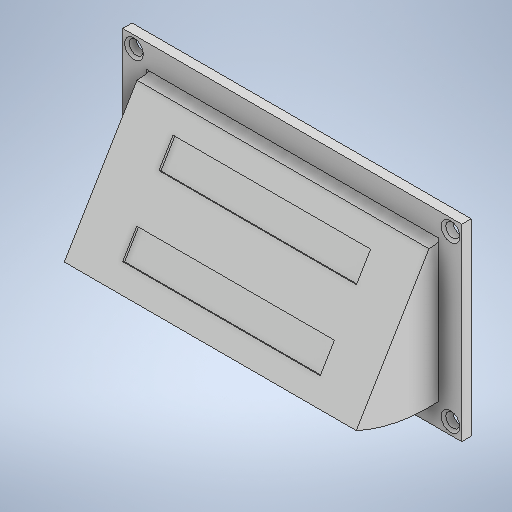
# Autodesk Inventor part: DsholdtilterV1
Saved by Autodesk Inventor 2025.1 (Build 291241000, 241)
## iProperties
Created: 2024-09-22
Part Number: DsholdtilterV1
Material: Generic
Document SubType Name: Modeling
Designer: ishaa
Density: 1 g/cm^3
Appearance: Default
Author: ishaa
Autodesk Inventor part; units mm, degrees
ref_plane "YZ Plane" through (0, 0, 0) normal (1, 0, 0) x (0, 1, 0)
ref_plane "XZ Plane" through (0, 0, 0) normal (0, 1, 0) x (-1, 0, 0)
ref_plane "XY Plane" through (0, 0, 0) normal (0, 0, 1) x (1, 0, 0)
sketch "Sketch1" plane through (0, 0, 0) normal (0, 0, 1) x (1, 0, 0)
  line L0 (0, 0) -> (62, 0)
  line L1 (62, 0) -> (62, 30)
  line L2 (62, 30) -> (0, 30)
  line L3 (0, 30) -> (0, 0)
  dimension "d0" = 62
  dimension "d1" = 30
  constraints: 8 end point, 2 parallel, 1 horizontal, 1 perpendicular
  measures "d0" distance of L2.end L1.end
  measures "d1" distance of L1.end L0.end
sketch "Sketch2" plane through (0, 0, 0) normal (1, 0, 0) x (0, 1, 0)
  line L0 (0, 0) -> (30, 0) projected
  arc A0 (16.1062, 11.6791) -> (15, 0) centre (36.6604, 3.8403) ccw
  constraints: 2 point on circle, 1 centre point, 1 midpoint
sweep "Sweep1" add profiles "Sketch1" path "Sketch2" path curves A0
sketch "Sketch3" plane through (62, 0, 0) normal (0, 0, -1) x (-1, 0, 0)
  line L0 (0, 0) -> (0, 30) projected
  line L1 (62, 0) -> (0, 0) projected
  line L2 (62, 30) -> (62, 0) projected
  line L3 (0, 30) -> (62, 30) projected
  line L4 (0, 30) -> (62, 0) construction
  line L5 (0, 0) -> (62, 30) construction
  line L6 (67, 35) -> (67, -5)
  line L7 (67, -5) -> (-5, -5)
  line L8 (-5, -5) -> (-5, 35)
  line L9 (-5, 35) -> (67, 35)
  dimension "d4" = 5
  constraints: 12 end point, 3 other
  measures "d4" distance between parallel lines of L3 L9
extrude "Extrusion1" add sketch "Sketch3" against normal blind 2
sketch "Sketch4" plane through (67, -5, 0) normal (0, 0, -1) x (-1, 0, 0)
  point P0 (67, 5)
sketch "Sketch6" plane through (0, 28.9732, 3.9694) normal (0, 0.514, 0.8578) x (1, 0, 0)
  line L0 (0, 1.893) -> (62, 1.893) construction
  line L1 (62, -30) -> (62, 0) construction
  line L2 (62, -15) -> (0, -15) construction
  line L3 (0, -23.9737) -> (0, -30) construction
  line L4 (31, -15) -> (31, -30) construction
  line L5 (31, -15) -> (31, 0) construction
  line L6 (62, 0) -> (0, 0) construction
  line L7 (62, -22.5) -> (31, -22.5) construction
  line L8 (31, -22.5) -> (0, -22.5) construction
  line L9 (31, -7.5) -> (0, -7.5) construction
  line L10 (0, 0) -> (0, -30) construction
  line L11 (31, -7.5) -> (62, -7.5) construction
  line L12 (51.9742, -19.576) -> (10.0258, -19.576)
  line L13 (10.0258, -19.576) -> (10.0258, -25.424)
  line L14 (10.0258, -25.424) -> (51.9742, -25.424)
  line L15 (51.9742, -25.424) -> (51.9742, -19.576)
  line L16 (51.9742, -19.576) -> (10.0258, -25.424) construction
  line L17 (10.0258, -19.576) -> (51.9742, -25.424) construction
  line L18 (51.9742, -10.424) -> (10.0258, -10.424)
  line L19 (10.0258, -10.424) -> (10.0258, -4.576)
  line L20 (10.0258, -4.576) -> (51.9742, -4.576)
  line L21 (51.9742, -4.576) -> (51.9742, -10.424)
  point P0 (0, -22.8131)
  dimension "d8" = 15
  dimension "d9" = 15
  dimension "d10" = 82.064
  dimension "d11" = 41.9483
  constraints: 34 end point, 7 midpoint, 7 point on line, 4 symmetric about line, 3 parallel, 2 horizontal, 1 perpendicular, 1 vertical
  measures "d8" distance between parallel lines of L8 L11
  measures "d9" distance of L7.start L11.end
  measures "d10" angle of L16 L15
  measures "d11" distance between parallel lines of L13 L15
extrude "Extrusion2" cut sketch "Sketch6" against normal blind 0.5
sketch "Sketch7" plane through (67, -5, 0) normal (0, 0, -1) x (-1, 0, 0)
  circle A0 centre (2.3883, 37.4725) radius 1.5
  line L0 (72, 40) -> (0, 40) construction
  line L1 (36, 40) -> (36, 0) construction
  line L2 (72, 0) -> (0, 0) construction
  line L3 (0, 40) -> (0, 0) construction
  line L4 (0, 20) -> (72, 20) construction
  line L5 (72, 40) -> (72, 0) construction
  circle A1 centre (2.3883, 2.5275) radius 1.5
  circle A2 centre (69.6117, 37.4725) radius 1.5
  circle A3 centre (69.6117, 2.5275) radius 1.5
  point P0 (67, 5)
  dimension "d14" = 3
  constraints: 4 centre point, 4 end point, 4 midpoint, 3 symmetric about line, 3 other
  measures "d14" diameter of A0
extrude "Extrusion3" cut sketch "Sketch7" against normal blind 25.4
chamfer "Chamfer1" distance 0.5 angle 45 4 edges at (-1.1117, -2.4725, 2) (66.1117, -2.4725, 2) (66.1117, 32.4725, 2) (-1.1117, 32.4725, 2)
body "Solid1"
